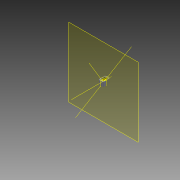
# Autodesk Inventor part: LED2
Saved by Autodesk Inventor 2011 SP2 (Build 150309200, 309)
## iProperties
Created: 2011-11-10
Part Number: LED2
Document SubType Name: Modeling
Designer: sungwook
Density: 1 g/cm^3
Author: sungwook
Autodesk Inventor part; units mm, degrees
ref_plane "YZ Plane" through (0, 0, 0) normal (1, 0, 0) x (0, 1, 0)
ref_plane "XZ Plane" through (0, 0, 0) normal (0, 1, 0) x (-1, 0, 0)
ref_plane "XY Plane" through (0, 0, 0) normal (0, 0, 1) x (1, 0, 0)
sketch "Sketch1" plane through (0, 0, 0) normal (0, 0, 1) x (1, 0, 0)
  line L0 (-0.75, 1.15) -> (0.75, 1.15)
  line L1 (0.75, 1.15) -> (0.75, -1.15)
  line L2 (0.75, -1.15) -> (-0.75, -1.15)
  line L3 (-0.75, -1.15) -> (-0.75, 1.15)
  point P0 (0, 0)
  point P1 (0, 1.15)
  point P2 (-0.75, 0)
  dimension "d0" = 1.5
  dimension "d1" = 2.3
  constraints: 8 end point, 2 midpoint, 2 parallel, 1 horizontal, 1 horizontal alignment, 1 perpendicular, 1 vertical alignment
  measures "d0" distance between parallel lines of L1 L3
  measures "d1" distance of L0.end L1.end
extrude "Extrusion1" add sketch "Sketch1" along normal blind 1.4
sketch "Sketch2" plane through (0, 0, 0) normal (0, 0, -1) x (-1, 0, 0)
  line L0 (0.75, 1.15) -> (-0.75, 1.15) projected
  line L1 (-0.75, 1.15) -> (-0.75, -1.15) projected
  line L2 (-0.75, -1.15) -> (0.75, -1.15) projected
  line L3 (0.75, -1.15) -> (0.75, 1.15) projected
  line L4 (-1.4, 1.5) -> (1.4, 1.5)
  line L5 (1.4, 1.5) -> (1.4, -1.5)
  line L6 (1.4, -1.5) -> (-1.4, -1.5)
  line L7 (-1.4, -1.5) -> (-1.4, 1.5)
  point P0 (0, 0)
  point P1 (-1.4, 0)
  point P2 (0, 1.5)
  dimension "d4" = 2.8
  dimension "d5" = 3
  constraints: 8 end point, 2 midpoint, 2 parallel, 1 horizontal, 1 horizontal alignment, 1 perpendicular, 1 vertical alignment
  measures "d4" distance between parallel lines of L5 L7
  measures "d5" distance between parallel lines of L6 L4
extrude "Extrusion2" [suppressed]
sketch "Sketch3" plane through (0, 0, 1.4) normal (0, 0, 1) x (1, 0, 0)
  line L0 (0.75, 1.15) -> (0.75, -1.15) projected
  line L1 (-0.75, 1.15) -> (0.75, 1.15) projected
  line L2 (-0.75, -1.15) -> (-0.75, 1.15) projected
  line L3 (0.75, -1.15) -> (-0.75, -1.15) projected
  line L4 (-0.5, 1.15) -> (0.5, 1.15)
  line L5 (0.5, 1.15) -> (0.5, -1.15)
  line L6 (0.5, -1.15) -> (-0.5, -1.15)
  line L7 (-0.5, -1.15) -> (-0.5, 1.15)
  line L8 (-0.75, 0.95) -> (0.75, 0.95)
  line L9 (0.75, 0.95) -> (0.75, -0.95)
  line L10 (0.75, -0.95) -> (-0.75, -0.95)
  line L11 (-0.75, -0.95) -> (-0.75, 0.95)
  line L12 (-0.75, 1.15) -> (-0.5, 1.15)
  line L13 (-0.5, 1.15) -> (-0.5, 0.95)
  line L14 (-0.5, 0.95) -> (-0.75, 0.95)
  line L15 (-0.75, 0.95) -> (-0.75, 1.15)
  point P0 (0, 0)
  point P1 (0, 1.15)
  point P2 (-0.75, 0)
  dimension "d8" = 1
  dimension "d9" = 1.9
  constraints: 24 end point, 6 parallel, 6 point on line, 3 horizontal, 3 perpendicular, 2 midpoint, 1 horizontal alignment, 1 vertical alignment
  measures "d8" distance between parallel lines of L5 L7
  measures "d9" distance between parallel lines of L10 L8
extrude "Extrusion3" [suppressed]
pattern_of_nothing "Mirror1"
pattern_of_nothing "Mirror2"
sketch "Sketch4" plane through (0, 0, 1.4) normal (0, 0, 1) x (1, 0, 0)
  line L0 (-0.5, 0.75) -> (0.5, 0.75)
  line L1 (0.5, 0.75) -> (0.5, -0.75)
  line L2 (0.5, -0.75) -> (-0.5, -0.75)
  line L3 (-0.5, -0.75) -> (-0.5, 0.75)
  point P0 (0, 0)
  point P1 (-0.5, 0)
  point P2 (0, 0.75)
  dimension "d12" = 1
  dimension "d13" = 1.5
  constraints: 8 end point, 2 midpoint, 2 parallel, 1 horizontal, 1 horizontal alignment, 1 perpendicular, 1 vertical alignment
  measures "d12" distance between parallel lines of L1 L3
  measures "d13" distance between parallel lines of L2 L0
extrude "Extrusion4" cut sketch "Sketch4" against normal blind 1 draft -10
sketch "Sketch5" plane through (0, 0, 0.4) normal (0, 0, 1) x (1, 0, 0)
  line L0 (-0.15, -0.1) -> (0.15, -0.1)
  line L1 (0.15, -0.1) -> (0.15, -0.4238)
  line L2 (0.15, -0.4238) -> (-0.15, -0.4238)
  line L3 (-0.15, -0.4238) -> (-0.15, -0.1)
  line L4 (-1.05, 0) -> (1.05, 0) projected
  point P0 (0, 0)
  point P1 (0, -0.1)
  dimension "d16" = 0.1
  dimension "d17" = 0.3
  dimension "d18" = 0.3
  constraints: 8 end point, 2 parallel, 1 horizontal, 1 midpoint, 1 perpendicular, 1 vertical alignment
  measures "d16" distance between parallel lines of L4 L0
  measures "d17" distance between parallel lines of L1 L3
  measures "d18" distance of L1.end L2.end
extrude "Extrusion5" add sketch "Sketch5" along normal blind 0.2
sketch "Sketch6" plane through (0, 0, 0.6) normal (0, 0, 1) x (1, 0, 0)
  line L0 (-0.15, -0.1) -> (0.15, -0.1) projected
  line L1 (-0.15, -0.4238) -> (-0.15, -0.1) projected
  circle A0 centre (0, -0.2619) radius 0.1
  line L2 (-1.05, 0) -> (1.05, 0) projected
  point P0 (0, 0)
  point P1 (0, -0.1)
  point P2 (-0.15, -0.2619)
  dimension "d21" = 0.2
  dimension "d24" = 0.2619
  constraints: 2 midpoint, 1 centre point, 1 coincident, 1 horizontal alignment, 1 vertical alignment
  measures "d21" diameter of A0
  measures "d24" distance from line of L2 A0.centre
extrude "Extrusion6" add sketch "Sketch6" along normal blind 0.05
extrude "Extrusion7" cut sketch "Sketch3" against normal through all contours L7 L8 L2 L1
pattern_linear "Rectangular Pattern1" count 2 spacing 1.5 along (1, 0, 0) count 2 spacing 2.3 along (0, 1, 0) of "Extrusion7"
mirror "Mirror3" about plane through (0, 0, 0) normal (-1, 0, 0) of "Extrusion7"
mirror "Mirror4" about plane through (0, 0, 0) normal (0, 1, 0) of "Extrusion7", "Mirror3"
sketch "Sketch8" plane through (0, 0, 1.4) normal (0, 0, 1) x (1, 0, 0)
  line L0 (0.5, -0.95) -> (0.75, -0.95) projected
  line L1 (0.75, 0.95) -> (0.75, -0.95) projected
  line L2 (0.75, 0.95) -> (0.5, 0.95) projected
  line L3 (0.5, 0.95) -> (0.5, 1.15) projected
  line L4 (-0.5, 1.15) -> (0.5, 1.15) projected
  line L5 (-0.5, 1.15) -> (-0.5, 0.95) projected
  line L6 (-0.5, 0.95) -> (-0.75, 0.95) projected
  line L7 (-0.75, -0.95) -> (-0.75, 0.95) projected
  line L8 (-0.75, -0.95) -> (-0.5, -0.95) projected
  line L9 (-0.5, -0.95) -> (-0.5, -1.15) projected
  line L10 (0.5, -1.15) -> (-0.5, -1.15) projected
  line L11 (0.5, -1.15) -> (0.5, -0.95) projected
  line L12 (-0.5, -0.75) -> (-0.5, 0.75) projected
  line L13 (-0.5, 0.75) -> (0.5, 0.75) projected
  line L14 (0.5, 0.75) -> (0.5, -0.75) projected
  line L15 (0.5, -0.75) -> (-0.5, -0.75) projected
  point P0 (0, 0)
  point P1 (0, -0.75)
  constraints: 1 midpoint
ref_plane "Work Plane1" through (0, 0, 0) normal (1, 0, 0) x (0, 1, 0)
ref_plane "Work Plane2" through (0, 0, 0) normal (-1, 0, 0) x (0, -1, 0)
ref_plane "Work Plane3" through (0, 0, 0) normal (-1, 0, 0) x (0, -1, 0)
ref_plane "Work Plane4" through (0, 0, 0) normal (0, 1, 0) x (-1, 0, 0)
ref_plane "Work Plane5" through (0, -0.2619, 0.6) normal (0, -1, 0) x (1, 0, 0)
body "Solid1"
